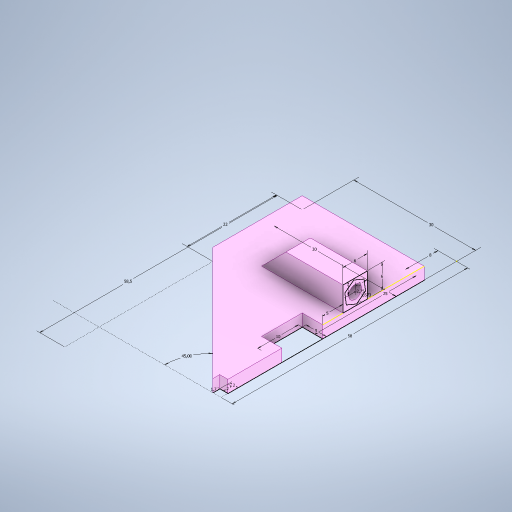
# Autodesk Inventor part: ScianaBocznaPEMv2
Saved by Autodesk Inventor 2023 (Build 270158000, 158)
## iProperties
Created: 2023-02-16
Part Number: ScianaBocznaPEMv2
Material: Generic
Document SubType Name: Modeling
Designer: KMRro
Density: 1 g/cm^3
Appearance: Default
Author: KMRro
Autodesk Inventor part; units mm, degrees
ref_plane "YZ Plane" through (0, 0, 0) normal (1, 0, 0) x (0, 1, 0)
ref_plane "XZ Plane" through (0, 0, 0) normal (0, 1, 0) x (-1, 0, 0)
ref_plane "XY Plane" through (0, 0, 0) normal (0, 0, 1) x (1, 0, 0)
sketch "Szkic1" plane through (0, 0, 0) normal (0, 1, 0) x (-1, 0, 0)
  line L0 (0, 8) -> (0, 56.3)
  line L1 (0, 58) -> (2, 58) construction
  line L2 (2, 58) -> (2, 56.3) construction
  line L3 (2, 56.3) -> (0, 56.3) construction
  line L4 (0, 56.3) -> (0, 58) construction
  line L5 (30, 8) -> (30, 66.5) construction
  line L6 (2, 58) -> (30, 30)
  line L7 (2, 58) -> (41.598, 58) construction
  line L8 (30, 30) -> (30, 8)
  line L9 (2, 58) -> (2, 56.3)
  line L10 (0, 56.3) -> (2, 56.3)
  line L11 (2, 56.3) -> (2, 54.3) construction
  line L12 (0, 43) -> (5, 43)
  line L13 (5, 43) -> (5, 33)
  line L14 (5, 33) -> (0, 33)
  line L15 (0, 33) -> (0, 43)
  line L16 (30, 8) -> (0, 8)
  line L17 (30, 8) -> (30, 30)
  point P0 (0, 0)
  point P1 (0, 33)
  dimension "d0" = 58
  dimension "d1" = 2
  dimension "d2" = 1.7
  dimension "d4" = 45
  dimension "d7" = 2
  dimension "d8" = 5
  dimension "d9" = 10
  dimension "d13" = 30
  dimension "d14" = 22
  dimension "d15" = 58.5
  dimension "d16" = 30
  dimension "d17" = 25
  dimension "d18" = 8
  constraints: 36 end point, 4 parallel, 4 perpendicular, 3 collinear, 3 horizontal, 2 point on line, 2 vertical, 1 equal length
  measures "d0" distance of point (0, 0) L1.start
  measures "d1" distance of L0.end L2.end
  measures "d2" distance of L1.end L2.end
  measures "d4" angle of L6 L7
  measures "d7" distance of L2.end L11.end
  measures "d8" distance of L13.end L14.end
  measures "d9" distance of L12.end L13.end
  measures "d13" distance of L5.start L0.start
  measures "d14" distance of L6.end L5.start
  measures "d15" distance of L5.start L5.end
  measures "d16" distance from line of point (0, 0) L5
  measures "d17" distance between parallel lines of L16 L14
  measures "d18" distance from line of point (0, 0) L16
extrude "Wyciągnięcie proste1" add sketch "Szkic1" along normal blind 3
extrude "Wyciągnięcie proste2" cut sketch "Szkic1" along normal blind 10 contours L0 L12 L13 L14
sketch "Sketch2" plane through (0, 0, 8) normal (1, 0, 0) x (0, 0, -1)
  line L0 (-25, 3) -> (0, 3) projected
  line L1 (-20, 3) -> (-14, 3)
  line L2 (-14, 3) -> (-14, 9)
  line L3 (-14, 9) -> (-20, 9)
  line L4 (-20, 9) -> (-20, 3)
  line L5 (-14.4598, 4.9465) -> (-16.6422, 3.2734)
  line L6 (-16.6422, 3.2734) -> (-19.1824, 4.3268)
  line L7 (-19.1824, 4.3268) -> (-19.5402, 7.0535)
  line L8 (-19.5402, 7.0535) -> (-17.3578, 8.7266)
  line L9 (-17.3578, 8.7266) -> (-14.8176, 7.6732)
  line L10 (-14.8176, 7.6732) -> (-14.4598, 4.9465)
  point P0 (8, 0)
  point P1 (-17, 6)
  point P2 (-17, 6)
  dimension "d19" = 6
  dimension "d20" = 6
  dimension "d21" = 5
  dimension "d24" = 3
  dimension "d25" = 3
  dimension "d29" = 1.6731
  dimension "d30" = 2.75
  constraints: 20 end point, 2 parallel, 1 coincident, 1 horizontal, 1 perpendicular, 1 point on line, 13 other
  measures "d19" distance of L3.end L2.end
  measures "d20" distance of L2.end L1.end
  measures "d21" distance of L0.start L1.start
  measures "d24" distance from line of L2 point (-17, 6)
  measures "d25" distance from line of L3 point (-17, 6)
  measures "d29" vertical distance of L5.start L5.end
  measures "d30" distance of L5.start point (-17, 6)
extrude "Extrusion3" add sketch "Sketch2" against normal blind 20 contours L4 L3 L2 L0 | L5 L6 L7 L8 L9 L10
extrude "Extrusion4" cut sketch "Sketch2" along normal blind 6 from surface at -20 contours L5 L6 L7 L8 L9 L10
chamfer "Chamfer2" distance 6 angle 45 1 edges at (-20, 9, 25)
hole "Hole1" at (0, 6, 25) direction (-1, 0, 0) diameter 3.2 depth 30 clearance for "Countersunk Flat Head Screw ISO 2009/7046" size "M3" standard "ISO"
